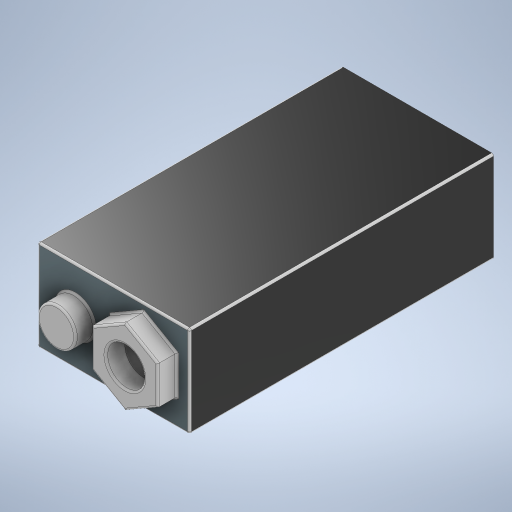
# Autodesk Inventor part: SPARC BOT Battery
Saved by Autodesk Inventor 2024 (Build 280153000, 153)
## iProperties
Created: 2023-07-01
Part Number: SPARC BOT Battery
Material: Generic
Document SubType Name: Modeling
Designer: Asus
Density: 1 g/cm^3
Appearance: Default
Author: Asus
Autodesk Inventor part; units mm, degrees
ref_plane "YZ Plane" through (0, 0, 0) normal (1, 0, 0) x (0, 1, 0)
ref_plane "XZ Plane" through (0, 0, 0) normal (0, 1, 0) x (-1, 0, 0)
ref_plane "XY Plane" through (0, 0, 0) normal (0, 0, 1) x (1, 0, 0)
sketch "Sketch1" plane through (0, 0, 0) normal (0, 0, 1) x (1, 0, 0)
  line L0 (20, 12) -> (0, 12)
  line L1 (0, 12) -> (0, 0)
  line L2 (0, 0) -> (20, 0)
  line L3 (20, 0) -> (20, 12)
  constraints: 8 end point, 2 parallel, 1 horizontal, 1 perpendicular
extrude "Extrusion1" add sketch "Sketch1" along normal blind 40
sketch "Sketch2" plane through (0, 0, 40) normal (0, 0, 1) x (1, 0, 0)
  circle A0 centre (5, 6) radius 2.5
  line L0 (14, 1) -> (9.6699, 3.5)
  line L1 (9.6699, 3.5) -> (9.6699, 8.5)
  line L2 (9.6699, 8.5) -> (14, 11)
  line L3 (14, 11) -> (18.3301, 8.5)
  line L4 (18.3301, 8.5) -> (18.3301, 3.5)
  line L5 (18.3301, 3.5) -> (14, 1)
  point P0 (0, 0)
  point P1 (14, 6)
  constraints: 12 end point, 1 centre point, 13 other
extrude "Extrusion2" add sketch "Sketch2" along normal blind 2.5
sketch "Sketch3" plane through (0, 0, 42.5) normal (0, 0, 1) x (1, 0, 0)
  circle A0 centre (14, 6) radius 2.5
  point P0 (0, 0)
  dimension "d15" = 5
  constraints: 1 centre point
  measures "d15" diameter of A0
extrude "Extrusion3" cut sketch "Sketch3" against normal blind 2.5
fillet "Fillet1" radius 0.25 1 edges at (2.5, 6, 42.5)
fillet "Fillet2" radius 0.25 13 edges at (11.8349, 2.25, 42.5) (16.1651, 2.25, 42.5) (18.3301, 6, 42.5) (9.6699, 6, 42.5) (11.8349, 9.75, 42.5) (16.1651, 9.75, 42.5) (11.5, 6, 42.5) (16.1651, 2.25, 40) (11.8349, 2.25, 40) (18.3301, 6, 40) (16.1651, 9.75, 40) (9.6699, 6, 40) (11.8349, 9.75, 40)
fillet "Fillet3" radius 0.25 1 edges at (2.5, 6, 40)
fillet "Fillet4" radius 0.25 8 edges at (20, 0, 20) (20, 12, 20) (0, 12, 20) (0, 0, 20) (0, 6, 40) (10, 0, 40) (20, 6, 40) (10, 12, 40)
body "Solid1"
